rod_label_clip (Autodesk Fusion 360 design; units mm, degrees)
part number: 2026-09-05-07-00-16-324
Autodesk Fusion 360 part; units mm, degrees
sketch "Ring" plane through (0, 0, 0) normal (0, 1, 0) x (1, 0, 0)
  circle A0 centre (0, 0) radius 17.05
  circle A1 centre (0, 0) radius 19.45
  dimension "d91" = 34.1
  dimension "d92" = 38.9
  constraint coincident A0.centre A1.centre
  constraint concentric A0 A1
  measures "d91" diameter of A0
  measures "d92" diameter of A1
extrude "Ring (1)" add sketch "Ring" along normal mid plane 9
sketch "Mouth" plane through (0, 0, 0) normal (0, 1, 0) x (1, 0, 0)
  line L0 (0, 0) -> (42.3486, -24.45)
  line L1 (42.3486, -24.45) -> (0, -48.9)
  line L2 (0, -48.9) -> (-42.3486, -24.45)
  line L3 (-42.3486, -24.45) -> (0, 0)
  line L4 (0, 0) -> (0, -48.9) construction
  dimension "d95" = 48.9
  dimension "d96" = 48.9
  dimension "d97" = 48.9
  dimension "d98" = 60
  dimension "d99" = 60
  constraint coincident L0.start L3.end
  constraint vertical L4
  constraint coincident L1.end L2.start
  measures "d95" distance of L0.start L0.end
  measures "d96" distance of L0.start L2.end
  measures "d97" distance of L0.start L1.end
  measures "d98" angle of L0 L4
  measures "d99" angle of L3 L4
extrude "Mouth (1)" cut sketch "Mouth" along normal mid plane 19
sketch "Stem" plane through (0, 0, 0) normal (0, 1, 0) x (1, 0, 0)
  line L0 (11.2039, 11.4854) -> (20.8457, 22.976)
  line L1 (20.8457, 22.976) -> (19.0072, 24.5187)
  line L2 (19.0072, 24.5187) -> (9.3653, 13.0281)
  line L3 (9.3653, 13.0281) -> (11.2039, 11.4854)
  dimension "d102" = 11.2039
  dimension "d103" = 11.4854
  dimension "d104" = 20.8457
  dimension "d105" = 22.976
  dimension "d106" = 19.0072
  dimension "d107" = 24.5187
  dimension "d108" = 9.3653
  dimension "d109" = 13.0281
  measures "d102" horizontal distance of origin L0.start
  measures "d103" vertical distance of origin L0.start
  measures "d104" horizontal distance of origin L0.end
  measures "d105" vertical distance of origin L0.end
  measures "d106" horizontal distance of origin L1.end
  measures "d107" vertical distance of origin L1.end
  measures "d108" horizontal distance of origin L2.end
  measures "d109" vertical distance of origin L2.end
extrude "Stem (1)" add sketch "Stem" along normal mid plane 9
sketch "Label face" plane through (0, 0, 0) normal (0, 1, 0) x (1, 0, 0)
  line L0 (20.8457, 22.976) -> (39.4865, 45.1913)
  line L1 (39.4865, 45.1913) -> (37.648, 46.734)
  line L2 (37.648, 46.734) -> (19.0072, 24.5187)
  line L3 (19.0072, 24.5187) -> (20.8457, 22.976)
  dimension "d112" = 20.8457
  dimension "d113" = 22.976
  dimension "d114" = 39.4865
  dimension "d115" = 45.1913
  dimension "d116" = 37.648
  dimension "d117" = 46.734
  dimension "d118" = 19.0072
  dimension "d119" = 24.5187
  measures "d112" horizontal distance of origin L0.start
  measures "d113" vertical distance of origin L0.start
  measures "d114" horizontal distance of origin L0.end
  measures "d115" vertical distance of origin L0.end
  measures "d116" horizontal distance of origin L1.end
  measures "d117" vertical distance of origin L1.end
  measures "d118" horizontal distance of origin L2.end
  measures "d119" vertical distance of origin L2.end
extrude "Label face (1)" add sketch "Label face" along normal mid plane 58
equation "clipWidth = 9.0 mm" comment "ring and stem width along the rod"
equation "faceWidth = 58.0 mm" comment "label face width along the rod"
equation "rodOuterDiameter = 33.4 mm" comment "rod the clip snaps onto"
equation "clipClearance = 0.7 mm" comment "diametral, so the clip slides"
equation "clipWall = 2.4 mm" comment "ring wall thickness"
equation "mouthHalfAngleDeg = 60.0 deg" comment "half the mouth opening"
equation "paddleThickness = 2.4 mm" comment "stem and label face thickness"
equation "stemEndRadius = 31.0 mm" comment "stem ends, label face begins"
equation "faceEndRadius = 60.0 mm" comment "outer edge of the label face"
equation "paddleAngleDeg = 50.0 deg" comment "paddle drop below horizontal"
equation "stemStartRadius = 16.0 mm" comment "stem starts inside the ring"
equation "d91 = rodOuterDiameter + clipClearance"
equation "d92 = rodOuterDiameter + clipClearance + 2 * clipWall"
equation "d93 = clipWidth"
equation "d95 = ( ( rodOuterDiameter + clipClearance + 2 * clipWall ) / 2 + 5 mm ) / cos(mouthHalfAngleDeg)"
equation "d96 = ( ( rodOuterDiameter + clipClearance + 2 * clipWall ) / 2 + 5 mm ) / cos(mouthHalfAngleDeg)"
equation "d97 = ( ( rodOuterDiameter + clipClearance + 2 * clipWall ) / 2 + 5 mm ) / cos(mouthHalfAngleDeg)"
equation "d98 = mouthHalfAngleDeg"
equation "d99 = mouthHalfAngleDeg"
equation "d100 = clipWidth + 10 mm"
equation "d102 = stemStartRadius * cos(paddleAngleDeg) + paddleThickness / 2 * sin(paddleAngleDeg)"
equation "d103 = stemStartRadius * sin(paddleAngleDeg) - paddleThickness / 2 * cos(paddleAngleDeg)"
equation "d104 = stemEndRadius * cos(paddleAngleDeg) + paddleThickness / 2 * sin(paddleAngleDeg)"
equation "d105 = stemEndRadius * sin(paddleAngleDeg) - paddleThickness / 2 * cos(paddleAngleDeg)"
equation "d106 = stemEndRadius * cos(paddleAngleDeg) - paddleThickness / 2 * sin(paddleAngleDeg)"
equation "d107 = stemEndRadius * sin(paddleAngleDeg) + paddleThickness / 2 * cos(paddleAngleDeg)"
equation "d108 = stemStartRadius * cos(paddleAngleDeg) - paddleThickness / 2 * sin(paddleAngleDeg)"
equation "d109 = stemStartRadius * sin(paddleAngleDeg) + paddleThickness / 2 * cos(paddleAngleDeg)"
equation "d110 = clipWidth"
equation "d112 = stemEndRadius * cos(paddleAngleDeg) + paddleThickness / 2 * sin(paddleAngleDeg)"
equation "d113 = stemEndRadius * sin(paddleAngleDeg) - paddleThickness / 2 * cos(paddleAngleDeg)"
equation "d114 = faceEndRadius * cos(paddleAngleDeg) + paddleThickness / 2 * sin(paddleAngleDeg)"
equation "d115 = faceEndRadius * sin(paddleAngleDeg) - paddleThickness / 2 * cos(paddleAngleDeg)"
equation "d116 = faceEndRadius * cos(paddleAngleDeg) - paddleThickness / 2 * sin(paddleAngleDeg)"
equation "d117 = faceEndRadius * sin(paddleAngleDeg) + paddleThickness / 2 * cos(paddleAngleDeg)"
equation "d118 = stemEndRadius * cos(paddleAngleDeg) - paddleThickness / 2 * sin(paddleAngleDeg)"
equation "d119 = stemEndRadius * sin(paddleAngleDeg) + paddleThickness / 2 * cos(paddleAngleDeg)"
equation "d120 = faceWidth"
named bodies: "rod_label_clip"
